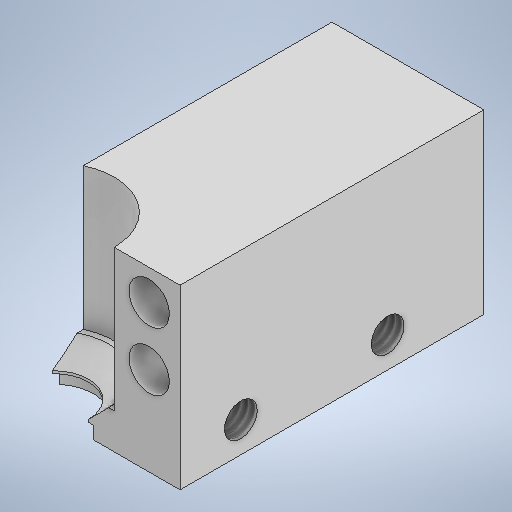
# Autodesk Inventor part: JH_int_Greiferkoerper
Saved by Autodesk Inventor 2025.2 (Build 292293000, 293)
## iProperties
Created: 2025-06-16
Part Number: JH_int_Greiferkoerper
Material: Generisch
Document SubType Name: Modeling
Designer: Jakob
Density: 1 g/cm^3
Appearance: Vorgabe
Author: Jakob
Autodesk Inventor part; units mm, degrees
ref_plane "YZ Plane" through (0, 0, 0) normal (1, 0, 0) x (0, 1, 0)
ref_plane "XZ Plane" through (0, 0, 0) normal (0, 1, 0) x (-1, 0, 0)
sketch "Skizze1" plane through (0, 0, 0) normal (0, 0, 1) x (1, 0, 0)
  line L0 (6.45, 0) -> (15, 0)
  line L1 (15, 0) -> (15, 30)
  line L2 (15, 30) -> (0, 30)
  line L3 (0, 30) -> (0, 3.0582)
  arc A0 (6.45, 0) -> (0, 3.0582) centre (2.5, 0) ccw
  line L4 (-3, 0) -> (18, 0) projected
  line L5 (0, -6) -> (0, 36) projected
  point P0 (0, 0)
  dimension "d0" = 30
  dimension "d1" = 15
  dimension "d2" = 7.9
  dimension "d3" = 2.5
  constraints: 8 end point, 2 parallel, 2 point on circle, 2 point on line, 1 centre point, 1 collinear, 1 horizontal, 1 perpendicular
  measures "d0" distance of L0.end L1.end
  measures "d1" distance of L1.end L2.end
  measures "d2" diameter of A0
  measures "d3" distance from line of L3 A0.centre
extrude "Extrusion1" add sketch "Skizze1" along normal mid plane 17.5 contours A0 L3 L2 L1 L0
ref_plane "Arbeitsebene1" through (0, 0, -7.5) normal (0, 0, 1) x (1, 0, 0)
sketch "Skizze2" plane through (0, 0, -7.5) normal (0, 0, 1) x (1, 0, 0)
  circle A0 centre (2.5, 0) radius 3.95
  arc A1 (6.45, 0) -> (0, 3.0582) centre (2.5, 0) ccw projected
  circle A2 centre (2.5, 0) radius 3.45
  line L0 (0, 3.0582) -> (0, 2.3775)
  line L1 (15, 0) -> (6.45, 0) projected
  line L2 (6.45, 0) -> (5.95, 0)
  point P0 (0, 0)
  point P1 (0, 3.0582)
  dimension "d7" = 7.9
  dimension "d8" = 6.9
  constraints: 4 end point, 2 centre point, 2 point on circle, 1 coincident, 1 collinear, 1 concentric, 1 vertical
  measures "d7" diameter of A0
  measures "d8" diameter of A2
extrude "Extrusion2" add sketch "Skizze2" along normal up to surface (16.25 mm away) contours L2 A2 L0 A0 picked at (6.25, 0.2945)
sketch "Skizze3" plane through (15, 0, 8.75) normal (1, 0, 0) x (0, 0, -1)
  line L0 (17.5, 30) -> (17.5, 0) projected
  line L1 (-3.5, 0) -> (21, 0) projected
  point P0 (8.75, 0)
  point P1 (14.5, 20.5)
  point P2 (14.5, 6)
  dimension "d11" = 3
  dimension "d12" = 3
  dimension "d13" = 6
  dimension "d14" = 14.5
  measures "d11" distance from line of L0 point (14.5, 6)
  measures "d12" distance from line of L0 point (14.5, 20.5)
  measures "d13" distance from line of point (14.5, 6) L1
  measures "d14" distance of point (14.5, 20.5) point (14.5, 6)
hole "Bohrung1" at (15, 20.5, -5.75) at (15, 6, -5.75) direction (-1, 0, 0) diameter 3.242 depth 8 tip angle 118 thread size "M4x0.7" class "6H" standard "ISO Metric profile"
sketch "Skizze4" plane through (6.45, 0, -8.75) normal (0, -1, 0) x (1, 0, 0)
  line L0 (-9.45, 8.75) -> (11.55, 8.75) projected
  line L1 (8.55, 0) -> (8.55, 17.5) projected
  line L2 (8.55, 17.5) -> (-0.5, 17.5) projected
  line L3 (-6.45, 21) -> (-6.45, -3.5) projected
  point P0 (-6.45, 8.75)
  point P1 (5.5, 14.5)
  point P2 (5.5, 8.75)
  dimension "d24" = 3
  dimension "d35" = 11.95
  constraints: 1 point on line, 1 vertical alignment
  measures "d24" distance from line of L2 point (5.5, 14.5)
  measures "d35" distance from line of point (5.5, 14.5) L3
hole "Bohrung2" at (11.95, 0, 5.75) at (11.95, 0, 0) direction (0, 1, 0) diameter 4 depth 6 tip angle 118
sketch "Skizze5" plane through (0, 0, 8.75) normal (0, 0, 1) x (1, 0, 0)
  circle A0 centre (2.5, 0) radius 6
  arc A1 (5.95, 0) -> (0, 2.3775) centre (2.5, 0) ccw projected
  line L0 (0, 2.3775) -> (0, 5.4544)
  line L1 (5.95, 0) -> (8.5, 0)
  line L2 (15, 0) -> (5.95, 0) projected
  point P0 (0, 0)
  dimension "d32" = 12
  constraints: 4 end point, 2 point on circle, 1 centre point, 1 concentric, 1 point on line, 1 vertical
  measures "d32" diameter of A0
extrude "Extrusion3" cut sketch "Skizze5" against normal blind 14 contours L1 A1 L0 A0 picked at (7.6008, 0.4409)
chamfer "Fasen1" distance 2 angle 45 1 edges at (3.7801, 3.2037, -5.25)
sketch "Skizze6" plane through (0, 30, 8.75) normal (0, 1, 0) x (1, 0, 0)
  line L0 (0, 17.5) -> (15, 17.5) projected
  line L1 (0, 17.5) -> (0, 0) projected
  point P0 (0, 8.75)
  point P1 (10, 5)
  point P2 (10, 13)
  point P3 (3, 9)
  dimension "d39" = 4.5
  dimension "d40" = 12.5
  dimension "d41" = 8.5
  dimension "d42" = 10
  dimension "d43" = 3
  constraints: 1 vertical alignment
  measures "d39" distance from line of L0 point (10, 13)
  measures "d40" distance from line of L0 point (10, 5)
  measures "d41" distance from line of L0 point (3, 9)
  measures "d42" distance from line of L1 point (10, 13)
  measures "d43" distance from line of L1 point (3, 9)
hole "Bohrung3" at (10, 30, 3.75) at (10, 30, -4.25) direction (0, -1, 0) diameter 2.459 depth 6 tip angle 118 thread size "M3x0.5" class "6H" standard "ISO Metric profile"
hole "Bohrung4" at (3, 30, -0.25) direction (0, -1, 0) diameter 3 depth 5 tip angle 118
equation "\"d0\" = Laenge_Grundkoerper"
equation "\"d1\" = Breite_Grundkoerper"
equation "\"d2\" = D_Scheibe"
equation "\"d3\" = Abstand_D_Scheibe"
equation "\"d4\" = Tiefe_Grundkoerper"
equation "\"d7\" = D_Scheibe"
equation "\"d9\" = Tiefe_Grundkoerper"
equation "\"d11\" = Abstand_Bohrungen_y"
equation "\"d12\" = Abstand_Bohrungen_y"
equation "\"d13\" = Abstand_Bohrungen_x"
equation "\"d14\" = Abstand_Bohrungen"
equation "\"d24\" = Zentrierbohrung_y"
equation "\"d25\" = D_Zentrierbohrung"
equation "\"d30\" = T_Zentrierbohrung"
equation "\"Laenge_Grundkoerper\" = 30"
equation "\"Breite_Grundkoerper\" = 15"
equation "\"D_Scheibe\" = 7.9"
equation "\"Abstand_D_Scheibe\" = 2.5"
equation "\"Abstand_Arbeitsebene\" = 2"
equation "\"Tiefe_Grundkoerper\" = 17.5"
equation "\"Abstand_Bohrungen_y\" = 3"
equation "\"Abstand_Bohrungen_x\" = 6"
equation "\"Abstand_Bohrungen\" = 14.5"
equation "\"Zentrierbohrung_x\" = 6"
equation "\"D_Zentrierbohrung\" = 4"
equation "\"T_Zentrierbohrung\" = 6"
equation "\"Zentrierbohrung_y\" = 3"
